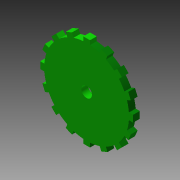
# Autodesk Inventor part: Motor Gear
Saved by Autodesk Inventor 2015 (Build 190159000, 159)
## iProperties
Created: 2018-02-28
Part Number: Motor Gear
Material: ABS Plastic
Document SubType Name: Modeling
Designer: Administrator
Density: 1.06 g/cm^3
Appearance: Dark Green
Author: Administrator
Autodesk Inventor part; units mm, degrees
ref_plane "YZ Plane" through (0, 0, 0) normal (1, 0, 0) x (0, 1, 0)
ref_plane "XZ Plane" through (0, 0, 0) normal (0, 1, 0) x (-1, 0, 0)
ref_plane "XY Plane" through (0, 0, 0) normal (0, 0, 1) x (1, 0, 0)
sketch "Sketch1" plane through (0, 0, 0) normal (0, 0, 1) x (1, 0, 0)
  circle A0 centre (0, 0) radius 8.001
  line L0 (-0.635, 8.763) -> (0.635, 8.763)
  line L1 (0.635, 8.763) -> (0.635, 7.9758)
  line L2 (-0.635, 7.9758) -> (-0.635, 8.763)
  circle A1 centre (0, 0) radius 1.0033
  dimension "d0" = 0.762
  dimension "d2" = 0.635
  dimension "d3" = 0.635
  dimension "d4" = 16.002
  dimension "d5" = 2.0066
  constraints: 6 end point, 2 centre point, 2 coincident, 2 point on circle, 1 horizontal, 1 parallel, 1 perpendicular
  measures "d0" distance edge to line of A0 L0
  measures "d2" distance from line of A0.centre L2
  measures "d3" distance from line of A0.centre L1
  measures "d4" diameter of A0
  measures "d5" diameter of A1
extrude "Extrusion1" add sketch "Sketch1" along normal mid plane 1.27 contours A0
extrude "Extrusion2" add sketch "Sketch1" along normal mid plane 1.27 contours A0 L2 L0 L1
pattern_circular "Circular Pattern1" count 16 over 360 about axis through (0, 0, 0) along (0, 0, 1) of "Extrusion2"
body "Solid1"
